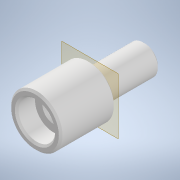
# Autodesk Inventor part: korek
Saved by Autodesk Inventor 2021 (Build 250183000, 183)
## iProperties
Created: 2021-05-20
Part Number: korek
Material: Polietylen, o małej gęstości
Document SubType Name: Modeling
Designer: Wojciech Wołczek
Density: 0.894 g/cm^3
Appearance: Gładki — w kolorze złamanej bieli
Author: Wojciech Wołczek
Autodesk Inventor part; units mm, degrees
ref_plane "YZ Plane" through (0, 0, 0) normal (1, 0, 0) x (0, 1, 0)
ref_plane "XZ Plane" through (0, 0, 0) normal (0, 1, 0) x (-1, 0, 0)
ref_plane "XY Plane" through (0, 0, 0) normal (0, 0, 1) x (1, 0, 0)
ref_plane "Płaszczyzna konstrukcyjna1" through (0, 0, 0) normal (0, 0, 1) x (1, 0, 0)
sketch "Szkic1" plane through (0, 0, 0) normal (0, 0, 1) x (1, 0, 0)
  circle A0 centre (-10, 0) radius 10 projected
  circle A1 centre (-10, 0) radius 15
  circle A2 centre (-10, 0) radius 10
  circle A3 centre (-10, 0) radius 8 projected
  circle A4 centre (-10, 0) radius 8
  circle A5 centre (-10, 0) radius 2
  point P0 (0, 0)
  dimension "d0" = 4
  constraints: 4 centre point, 3 coincident, 1 concentric, 1 horizontal alignment, 2 other
  measures "d0" diameter of A5
extrude "Wyciągnięcie proste1" add sketch "Szkic1" against normal blind 30 contours A3
sketch "Szkic2" plane through (-10, 0, 0) normal (0, 0, 1) x (1, 0, 0)
  circle A0 centre (0, 0) radius 8 projected
  circle A1 centre (0, 0) radius 2 projected
  circle A2 centre (0, 0) radius 2 projected
  circle A3 centre (0, 0) radius 2
  circle A4 centre (0, 0) radius 14 projected
  circle A5 centre (0, 0) radius 14
  point P0 (10, 0)
  constraints: 2 centre point, 2 coincident, 1 concentric
extrude "Wyciągnięcie proste2" add sketch "Szkic2" along normal blind 30 contours A0 | A4
sketch "Szkic3" plane through (-10, 0, 30) normal (0, 0, 1) x (1, 0, 0)
  circle A0 centre (0, 0) radius 2 projected
  circle A1 centre (0, 0) radius 10
  point P0 (10, 0)
  dimension "d5" = 20
  constraints: 1 centre point, 1 coincident
  measures "d5" diameter of A1
extrude "Wyciągnięcie proste3" cut sketch "Szkic3" against normal blind 10
sketch "Szkic4" plane through (-10, 0, 20) normal (0, 0, 1) x (1, 0, 0)
  circle A0 centre (0, 0) radius 5
  point P0 (10, 0)
  dimension "d8" = 10
  constraints: 1 centre point
  measures "d8" diameter of A0
extrude "Wyciągnięcie proste4" cut sketch "Szkic4" against normal blind 20
chamfer "Faza1" distance 1 angle 45 5 edges at (-20, 0, 30) (-15, 0, 20) (-24, 0, 30) (-24, 0, 0) (-18, 0, -30)
